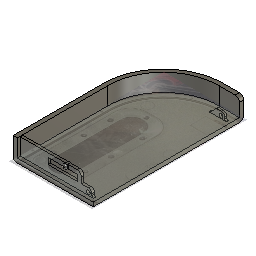
SD Card Door (Autodesk Fusion 360 design; units mm, degrees)
Autodesk Fusion 360 part; units mm, degrees
note: some values were not read from the file. Chosen so that the rebuilt part matches the saved one: which face or edge a step refers to; which pieces of a blend or face edit are solid.
sketch "initial square" plane through (0, 0, 0) normal (0, 0, 1) x (1, 0, 0)
  line L0 (0, 0) -> (-48, 0)
  line L1 (-48, 0) -> (-48, 90)
  line L2 (-48, 90) -> (0, 90)
  line L3 (0, 90) -> (0, 0)
  dimension "d1" = 48
  dimension "d2" = 90
  constraint horizontal L0
  constraint vertical L1
  constraint horizontal L2
  constraint vertical L3
  constraint coincident L0.start L3.end
  measures "d1" distance of L0.start L0.end
  measures "d2" distance of L0.start L2.end
sketch "part outline" plane through (0, 0, 0) normal (0, 0, 1) x (1, 0, 0)
  line L0 (-48, 90) -> (0, 90)
  line L1 (0, 90) -> (0, 0)
  line L2 (0, 90) -> (-12, 90)
  line L3 (-48, 0) -> (-48, 90) construction
  line L4 (-48, 54) -> (0, 54) construction
  line L5 (0, 0) -> (-48, 0) construction
  line L6 (-12, 90) -> (-12, 54) construction
  arc A0 (-12, 90) -> (-48, 54) centre (-12, 54) ccw
  line L7 (-48, 54) -> (-48, 0)
  line L8 (-48, 0) -> (0, 0)
  line L9 (0, 0) -> (0, 90)
  line L10 (-12, 87.5) -> (0, 87.5)
  line L11 (-45.5, 0) -> (-45.5, 54)
  arc A1 (-12, 87.5) -> (-45.5, 54) centre (-12.4838, 54.4838) ccw
  line L12 (-45.5, 3.5) -> (-2.8, 3.5)
  line L13 (-2.8, 3.5) -> (-2.8, 2)
  line L14 (-2.8, 2) -> (-45.5, 2)
  line L15 (-7.8, 82.7) -> (-2.8, 82.7)
  line L16 (-2.8, 82.7) -> (-2.8, 81.5)
  line L17 (-2.8, 81.5) -> (-7.8, 81.5)
  line L18 (-7.8, 81.5) -> (-7.8, 82.7)
  point P0 (0, 90)
  dimension "d7" = 36
  dimension "d8" = 36
  dimension "d11" = 2.5
  dimension "d12" = 2.5
  dimension "d13" = 1.5
  dimension "d14" = 2
  dimension "d15" = 2.8
  dimension "d16" = 5
  dimension "d17" = 1.2
  dimension "d18" = 2.8
  dimension "d19" = 78
  constraint coincident P0 L0.end
  constraint coincident L0 L2.end
  constraint coincident L3 L4.start
  constraint coincident L1 L4.end
  constraint perpendicular L1 L4
  constraint coincident L4 L6.end
  constraint perpendicular L4 L6
  constraint coincident L6.end A0.centre
  constraint coincident L3.start L5.end
  constraint coincident L1.end L5.start
  constraint coincident L1 L10.end
  constraint perpendicular L1 L10
  constraint coincident L8 L11.start
  constraint coincident L4 L11.end
  constraint coincident L6 L10.start
  constraint coincident L11 L12.start
  constraint perpendicular L11 L12
  constraint perpendicular L12 L13
  constraint coincident L11 L14.end
  constraint perpendicular L11 L14
  constraint horizontal L15
  constraint vertical L16
  constraint horizontal L17
  constraint vertical L18
  measures "d7" distance of L3 L6
  measures "d8" distance of L0 L4
  measures "d11" distance of L0 L10
  measures "d12" distance of L3 L11
  measures "d13" distance of L12.end L13.end
  measures "d14" distance of L5 L14
  measures "d15" distance of L1 L13
  measures "d16" distance of L15.start L15.end
  measures "d17" distance of L15.start L17.end
  measures "d18" distance of L1 L16
  measures "d19" distance of L12 L17
extrude "Extrude1" add sketch "part outline" along normal blind 13 contours L0 L1 L2 A0 L7 L8 L9 L10 L11 A1 makes body 1
extrude "Extrude2" add sketch "part outline" along normal blind 12.5 contours L11 L12 L13 L14 | L15 L16 L17 L18 bodies 1 makes body 2 at (-6.1333, 82.7, 4.1667)
sketch "latch and holes" plane through (0, 2, 0) normal (0, -1, 0) x (1, 0, 0)
  line L0 (-45.5, 0) -> (-2.8, 0)
  line L1 (-2.8, 0) -> (-2.8, 12.5)
  line L2 (-2.8, 12.5) -> (-45.5, 12.5)
  line L3 (-45.5, 12.5) -> (-45.5, 0)
  line L4 (-4, 12.5) -> (-4, 0) construction
  line L5 (0, 0) -> (0, 13) construction
  line L6 (-5, 0) -> (-5, 12.5) construction
  line L7 (-2.8, 3) -> (-45.5, 3) construction
  line L8 (-48, 0) -> (0, 0) construction
  line L9 (-4, 4) -> (-5, 4) construction
  circle A0 centre (-5, 4) radius 1.2
  line L10 (-29.1, 10.1) -> (-11.6, 10.1)
  line L11 (-11.6, 10.1) -> (-11.6, 6.4)
  line L12 (-11.6, 6.4) -> (-29.1, 6.4)
  line L13 (-29.1, 6.4) -> (-29.1, 10.1)
  line L14 (-9.1, 6.4) -> (-9.1, 12.5)
  line L15 (-9.1, 6.4) -> (-2.8, 6.4)
  line L16 (-18, 12.5) -> (-18, 10.1) construction
  line L17 (-48, 0) -> (-48, 13)
  circle A1 centre (-18, 11.3) radius 1.4
  dimension "d24" = 4
  dimension "d25" = 1
  dimension "d26" = 3
  dimension "d27" = 1
  dimension "d28" = 2.4
  dimension "d29" = 17.5
  dimension "d30" = 3.7
  dimension "d31" = 16.4
  dimension "d32" = 2.4
  dimension "d33" = 2.5
  dimension "d34" = 6.1
  dimension "d39" = 30
  dimension "d40" = 2.8
  constraint coincident L2 L4.start
  constraint coincident L0 L4.end
  constraint perpendicular L0 L4
  constraint coincident L0 L6.start
  constraint coincident L2 L6.end
  constraint perpendicular L2 L6
  constraint coincident L1 L7.start
  constraint coincident L3 L7.end
  constraint perpendicular L3 L7
  constraint coincident L4 L9.start
  constraint coincident L6 L9.end
  constraint perpendicular L6 L9
  constraint coincident L9.end A0.centre
  constraint horizontal L10
  constraint vertical L11
  constraint horizontal L12
  constraint vertical L13
  constraint coincident L2 L14.end
  constraint perpendicular L2 L14
  constraint coincident L1 L15.end
  constraint perpendicular L1 L15
  constraint coincident L2 L16.start
  constraint coincident L10 L16.end
  constraint perpendicular L10 L16
  constraint midpoint L16 A1.centre
  measures "d24" distance of L4 L5
  measures "d25" distance of L4 L6
  measures "d26" distance of L7 L8
  measures "d27" distance of L7 L9
  measures "d28" diameter of A0
  measures "d29" distance of L10.start L10.end
  measures "d30" distance of L10.start L12.end
  measures "d31" distance of L3 L13
  measures "d32" distance of L2 L10
  measures "d33" distance of L11 L14
  measures "d34" distance of L2 L15
  measures "d39" distance of L16 L17
  measures "d40" diameter of A1
extrude "Extrude3" cut sketch "latch and holes" against normal blind 80.7 contours L1 L2 L14 L15 | A0 bodies 1 2
extrude "Extrude4" cut sketch "latch and holes" against normal blind 1.5 contours L10 L11 L12 L13 A1 | L10 A1 bodies 1
extrude "Extrude5" add sketch "latch and holes" along normal blind 1.7 contours L2 A1 | L2 L10 A1 | L10 A1 bodies 1
extrude "Extrude6" add sketch "part outline" along normal blind 2.5 contours L1 L8 L9 L10 L11 A1 L12 L13 L14 bodies 1 2
fillet "Fillet1" radius 1 1 edges at (-19.3053, 0.3, 10.7937) on bodies 1
fillet "Fillet2" radius 2 2 edges at (-2.8, 2.75, 6.4) (-2.8, 82.1, 6.4) on bodies 1 2
chamfer "Chamfer1" distance 3.9 angle 45 1 edges at (-7.8, 82.1, 2.5) on bodies 1
fillet "Fillet3" radius 2.5 1 edges at (0, 88.75, 13) on bodies 1
fillet "Fillet4" radius 1 2 edges at (-2.8, 82.1, 2.5) (-2.8, 2.75, 2.5) on bodies 1
fillet "Fillet5" radius 1 5 edges at (-11.6992, 82.1, 2.5) (-7.8, 82.7, 6.3996) (-7.8, 82.1, 6.3992) (-7.8, 81.5, 6.3996) (-7.8, 82.1, 6.4) on bodies 1
fillet "Fillet6" radius 2.5 1 edges at (-9.1, 2.75, 12.5) on bodies 1
extrude "Extrude7" add 2 faces at (-18.1247, 2, 12.5497) (-18.1842, 2, 10.0712) along direction (0, 1, 0) blind 1.5 on bodies 1 bodies 1
fillet "Fillet7" radius 2.1 3 edges at (-6, 90, 0) (-37.4558, 79.4558, 0) (-48, 27, 0) on bodies 1
equation "d8 = d7"
equation "d9 = 2.5 mm"
equation "d12 = d11"
equation "d18 = d15"
equation "d22 = 13.00 mm - 0.5 mm"
equation "d25 = ( 2 / 2 ) * 1 mm"
equation "d27 = d25"
equation "d41 = 2.9 mm - 1.2 mm"
equation "d43 = d9"
named bodies: "SD Card Door"
